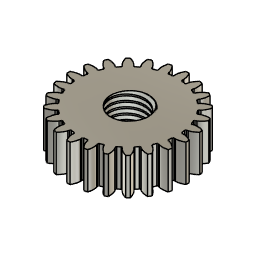
gear v1 (Autodesk Fusion 360 design; units mm, degrees)
description: Spur Gear; Module: 1.25; Num Teeth: 24; Pressure Angle: 20.0; Backlash: 0.00 mm
Autodesk Fusion 360 part; units mm, degrees
(part 1 of 3)
sketch "Sketch1" plane through (0, 0, 0) normal (0, 0, 1) x (1, 0, 0)
sketch "Sketch1 (2)" plane through (0, 0, 0) normal (0, 0, 1) x (1, 0, 0) in component "Spur Gear (24 teeth)"
  circle A0 centre (0, 0) radius 13.4492
extrude "Extrude1" add sketch "Sketch1 (2)" along normal blind 10 makes body 1 in component "Spur Gear (24 teeth)"
sketch "Sketch2" plane through (0, 0, 0) normal (0, 0, 1) x (1, 0, 0) in component "Spur Gear (24 teeth)"
  spline S0 degree 5 poles (14.0499, -1.1314) (14.0562, -1.1319) (14.0687, -1.1327) (14.0876, -1.1335) (14.1127, -1.1337) (14.1442, -1.1327) (14.1757, -1.1308) (14.2072, -1.1284) (14.2388, -1.1257) (14.2703, -1.1227) (14.3019, -1.1196) (14.3335, -1.1161) (14.3651, -1.1123) (14.3967, -1.1081) (14.4283, -1.1035) (14.4599, -1.0984) (14.4916, -1.093) (14.5232, -1.0873) (14.5548, -1.0814) (14.5864, -1.0752) (14.618, -1.0688) (14.6496, -1.0622) (14.6812, -1.0552) (14.7128, -1.048) (14.7444, -1.0406) (14.776, -1.0329) (14.8076, -1.0249) (14.8392, -1.0168) (14.8708, -1.0083) (14.9023, -0.9997) (14.9339, -0.9909) (14.9654, -0.9818) (14.997, -0.9725) (15.0285, -0.963) (15.06, -0.9533) (15.0915, -0.9434) (15.123, -0.9333) (15.1545, -0.923) (15.1859, -0.9124) (15.2174, -0.9017) (15.2488, -0.8908) (15.2802, -0.8797) (15.3116, -0.8684) (15.343, -0.8569) (15.3743, -0.8452) (15.4057, -0.8333) (15.437, -0.8213) (15.4683, -0.809) (15.4996, -0.7966) (15.5309, -0.784) (15.5621, -0.7712) (15.5934, -0.7583) (15.6246, -0.7451) (15.6558, -0.7318) (15.6869, -0.7183) (15.7181, -0.7047) (15.7492, -0.6909) (15.7803, -0.6769) (15.8114, -0.6627) (15.8425, -0.6484) (15.8735, -0.6339) (15.9045, -0.6192) (15.9355, -0.6044) (15.9664, -0.5894) (15.9974, -0.5742) (16.0283, -0.5589) (16.0592, -0.5434) (16.09, -0.5278) (16.1208, -0.512) (16.1516, -0.496) (16.1824, -0.4799) (16.207, -0.4669) (16.2254, -0.4571) (16.2377, -0.4505) (16.2438, -0.4472) knots 0 0 0 0 0 0 0.01428571 0.02857143 0.04285714 0.05714286 0.07142857 0.08571429 0.1 0.11428571 0.12857143 0.14285714 0.15714286 0.17142857 0.18571429 0.2 0.21428571 0.22857143 0.24285714 0.25714286 0.27142857 0.28571429 0.3 0.31428571 0.32857143 0.34285714 0.35714286 0.37142857 0.38571429 0.4 0.41428571 0.42857143 0.44285714 0.45714286 0.47142857 0.48571429 0.5 0.51428571 0.52857143 0.54285714 0.55714286 0.57142857 0.58571429 0.6 0.61428571 0.62857143 0.64285714 0.65714286 0.67142857 0.68571429 0.7 0.71428571 0.72857143 0.74285714 0.75714286 0.77142857 0.78571429 0.8 0.81428571 0.82857143 0.84285714 0.85714286 0.87142857 0.88571429 0.9 0.91428571 0.92857143 0.94285714 0.95714286 0.97142857 0.98571429 1 1 1 1 1 1
  spline S1 degree 5 poles (14.0499, 1.1314) (14.0562, 1.1319) (14.0687, 1.1327) (14.0876, 1.1335) (14.1127, 1.1337) (14.1442, 1.1327) (14.1757, 1.1308) (14.2072, 1.1284) (14.2388, 1.1257) (14.2703, 1.1227) (14.3019, 1.1196) (14.3335, 1.1161) (14.3651, 1.1123) (14.3967, 1.1081) (14.4283, 1.1035) (14.4599, 1.0984) (14.4916, 1.093) (14.5232, 1.0873) (14.5548, 1.0814) (14.5864, 1.0752) (14.618, 1.0688) (14.6496, 1.0622) (14.6812, 1.0552) (14.7128, 1.048) (14.7444, 1.0406) (14.776, 1.0329) (14.8076, 1.0249) (14.8392, 1.0168) (14.8708, 1.0083) (14.9023, 0.9997) (14.9339, 0.9909) (14.9654, 0.9818) (14.997, 0.9725) (15.0285, 0.963) (15.06, 0.9533) (15.0915, 0.9434) (15.123, 0.9333) (15.1545, 0.923) (15.1859, 0.9124) (15.2174, 0.9017) (15.2488, 0.8908) (15.2802, 0.8797) (15.3116, 0.8684) (15.343, 0.8569) (15.3743, 0.8452) (15.4057, 0.8333) (15.437, 0.8213) (15.4683, 0.809) (15.4996, 0.7966) (15.5309, 0.784) (15.5621, 0.7712) (15.5934, 0.7583) (15.6246, 0.7451) (15.6558, 0.7318) (15.6869, 0.7183) (15.7181, 0.7047) (15.7492, 0.6909) (15.7803, 0.6769) (15.8114, 0.6627) (15.8425, 0.6484) (15.8735, 0.6339) (15.9045, 0.6192) (15.9355, 0.6044) (15.9664, 0.5894) (15.9974, 0.5742) (16.0283, 0.5589) (16.0592, 0.5434) (16.09, 0.5278) (16.1208, 0.512) (16.1516, 0.496) (16.1824, 0.4799) (16.207, 0.4669) (16.2254, 0.4571) (16.2377, 0.4505) (16.2438, 0.4472) knots 0 0 0 0 0 0 0.01428571 0.02857143 0.04285714 0.05714286 0.07142857 0.08571429 0.1 0.11428571 0.12857143 0.14285714 0.15714286 0.17142857 0.18571429 0.2 0.21428571 0.22857143 0.24285714 0.25714286 0.27142857 0.28571429 0.3 0.31428571 0.32857143 0.34285714 0.35714286 0.37142857 0.38571429 0.4 0.41428571 0.42857143 0.44285714 0.45714286 0.47142857 0.48571429 0.5 0.51428571 0.52857143 0.54285714 0.55714286 0.57142857 0.58571429 0.6 0.61428571 0.62857143 0.64285714 0.65714286 0.67142857 0.68571429 0.7 0.71428571 0.72857143 0.74285714 0.75714286 0.77142857 0.78571429 0.8 0.81428571 0.82857143 0.84285714 0.85714286 0.87142857 0.88571429 0.9 0.91428571 0.92857143 0.94285714 0.95714286 0.97142857 0.98571429 1 1 1 1 1 1
  arc A0 (16.2438, -0.4472) -> (16.2438, 0.4472) centre (0, 0) ccw
  line L0 (13.3958, -1.0795) -> (14.0499, -1.1314)
  line L1 (13.3958, 1.0795) -> (14.0499, 1.1314)
  line L2 (13.3958, -1.0795) -> (13.3958, 1.0795)
  point P0 (14.2045, -1.1286)
  point P1 (14.3601, -1.1129)
  point P2 (14.5163, -1.0885)
  point P3 (14.673, -1.057)
  point P4 (14.8299, -1.0191)
  point P5 (14.9871, -0.9754)
  point P6 (15.1444, -0.9262)
  point P7 (15.3018, -0.8719)
  point P8 (15.4592, -0.8126)
  point P9 (15.6165, -0.7485)
  point P10 (15.7737, -0.6798)
  point P11 (15.9307, -0.6066)
  point P12 (16.0874, -0.5291)
  point P13 (14.2045, 1.1286)
  point P14 (14.3601, 1.1129)
  point P15 (14.5163, 1.0885)
  point P16 (14.673, 1.057)
  point P17 (14.8299, 1.0191)
  point P18 (14.9871, 0.9754)
  point P19 (15.1444, 0.9262)
  point P20 (15.3018, 0.8719)
  point P21 (15.4592, 0.8126)
  point P22 (15.6165, 0.7485)
  point P23 (15.7737, 0.6798)
  point P24 (15.9307, 0.6066)
  point P25 (16.0874, 0.5291)
extrude "Extrude2" add sketch "Sketch2" along normal blind 10 bodies 1 in component "Spur Gear (24 teeth)"
fillet "Fillet1" radius 0.25 2 edges at (13.4057, -1.0803, 5) (13.4057, 1.0803, 5) on bodies 1 in component "Spur Gear (24 teeth)"
pattern_circular "C-Pattern1" count 24 over 360 about axis through (0, 0, 0) along (0, 0, 1) of "Extrude2", "Fillet1" in component "Spur Gear (24 teeth)"
sketch "Sketch3" plane through (0, 0, 0) normal (0, 0, 1) x (1, 0, 0) in component "Spur Gear (24 teeth)"
  circle A0 centre (0, 0) radius 15 construction
copy_body "CopyPasteBodies1" bodies 1 makes body 2
move_body "Move1" bodies 2 to x (1, 0, 0) y (0, 1, 0) z (0, 0, 1) at (0, 40, 0)
sketch "Sketch2 (2)" plane through (0, 0, 10) normal (0, 0, 1) x (-1, 0, 0)
  arc A0 (-13.2706, -37.8154) -> (-13.3838, -38.6755) centre (0, -40) ccw
  arc A1 (-13.6524, -38.9001) -> (-13.3838, -38.6755) centre (-13.6326, -38.6509) ccw
  line L0 (-13.6524, -38.9001) -> (-14.0499, -38.8686)
  spline S0 degree 5 poles (-14.0499, -38.8686) (-14.0562, -38.8681) (-14.0687, -38.8673) (-14.0876, -38.8665) (-14.1127, -38.8663) (-14.1442, -38.8673) (-14.1757, -38.8692) (-14.2072, -38.8716) (-14.2388, -38.8743) (-14.2703, -38.8773) (-14.3019, -38.8804) (-14.3335, -38.8839) (-14.3651, -38.8877) (-14.3967, -38.8919) (-14.4283, -38.8965) (-14.4599, -38.9016) (-14.4916, -38.907) (-14.5232, -38.9127) (-14.5548, -38.9186) (-14.5864, -38.9248) (-14.618, -38.9312) (-14.6496, -38.9378) (-14.6812, -38.9448) (-14.7128, -38.952) (-14.7444, -38.9594) (-14.776, -38.9671) (-14.8076, -38.9751) (-14.8392, -38.9832) (-14.8708, -38.9917) (-14.9023, -39.0003) (-14.9339, -39.0091) (-14.9654, -39.0182) (-14.997, -39.0275) (-15.0285, -39.037) (-15.06, -39.0467) (-15.0915, -39.0566) (-15.123, -39.0667) (-15.1545, -39.077) (-15.1859, -39.0876) (-15.2174, -39.0983) (-15.2488, -39.1092) (-15.2802, -39.1203) (-15.3116, -39.1316) (-15.343, -39.1431) (-15.3743, -39.1548) (-15.4057, -39.1667) (-15.437, -39.1787) (-15.4683, -39.191) (-15.4996, -39.2034) (-15.5309, -39.216) (-15.5621, -39.2288) (-15.5934, -39.2417) (-15.6246, -39.2549) (-15.6558, -39.2682) (-15.6869, -39.2817) (-15.7181, -39.2953) (-15.7492, -39.3091) (-15.7803, -39.3231) (-15.8114, -39.3373) (-15.8425, -39.3516) (-15.8735, -39.3661) (-15.9045, -39.3808) (-15.9355, -39.3956) (-15.9664, -39.4106) (-15.9974, -39.4258) (-16.0283, -39.4411) (-16.0592, -39.4566) (-16.09, -39.4722) (-16.1208, -39.488) (-16.1516, -39.504) (-16.1824, -39.5201) (-16.207, -39.5331) (-16.2254, -39.5429) (-16.2377, -39.5495) (-16.2438, -39.5528) knots 0 0 0 0 0 0 0.01428571 0.02857143 0.04285714 0.05714286 0.07142857 0.08571429 0.1 0.11428571 0.12857143 0.14285714 0.15714286 0.17142857 0.18571429 0.2 0.21428571 0.22857143 0.24285714 0.25714286 0.27142857 0.28571429 0.3 0.31428571 0.32857143 0.34285714 0.35714286 0.37142857 0.38571429 0.4 0.41428571 0.42857143 0.44285714 0.45714286 0.47142857 0.48571429 0.5 0.51428571 0.52857143 0.54285714 0.55714286 0.57142857 0.58571429 0.6 0.61428571 0.62857143 0.64285714 0.65714286 0.67142857 0.68571429 0.7 0.71428571 0.72857143 0.74285714 0.75714286 0.77142857 0.78571429 0.8 0.81428571 0.82857143 0.84285714 0.85714286 0.87142857 0.88571429 0.9 0.91428571 0.92857143 0.94285714 0.95714286 0.97142857 0.98571429 1 1 1 1 1 1
  arc A2 (-16.2438, -39.5528) -> (-16.2438, -40.4472) centre (0, -40) ccw
  spline S1 degree 5 poles (-16.2438, -40.4472) (-16.2377, -40.4505) (-16.2254, -40.4571) (-16.207, -40.4669) (-16.1824, -40.4799) (-16.1516, -40.496) (-16.1208, -40.512) (-16.09, -40.5278) (-16.0592, -40.5434) (-16.0283, -40.5589) (-15.9974, -40.5742) (-15.9664, -40.5894) (-15.9355, -40.6044) (-15.9045, -40.6192) (-15.8735, -40.6339) (-15.8425, -40.6484) (-15.8114, -40.6627) (-15.7803, -40.6769) (-15.7492, -40.6909) (-15.7181, -40.7047) (-15.6869, -40.7183) (-15.6558, -40.7318) (-15.6246, -40.7451) (-15.5934, -40.7583) (-15.5621, -40.7712) (-15.5309, -40.784) (-15.4996, -40.7966) (-15.4683, -40.809) (-15.437, -40.8213) (-15.4057, -40.8333) (-15.3743, -40.8452) (-15.343, -40.8569) (-15.3116, -40.8684) (-15.2802, -40.8797) (-15.2488, -40.8908) (-15.2174, -40.9017) (-15.1859, -40.9124) (-15.1545, -40.923) (-15.123, -40.9333) (-15.0915, -40.9434) (-15.06, -40.9533) (-15.0285, -40.963) (-14.997, -40.9725) (-14.9654, -40.9818) (-14.9339, -40.9909) (-14.9023, -40.9997) (-14.8708, -41.0083) (-14.8392, -41.0168) (-14.8076, -41.0249) (-14.776, -41.0329) (-14.7444, -41.0406) (-14.7128, -41.048) (-14.6812, -41.0552) (-14.6496, -41.0622) (-14.618, -41.0688) (-14.5864, -41.0752) (-14.5548, -41.0814) (-14.5232, -41.0873) (-14.4916, -41.093) (-14.4599, -41.0984) (-14.4283, -41.1035) (-14.3967, -41.1081) (-14.3651, -41.1123) (-14.3335, -41.1161) (-14.3019, -41.1196) (-14.2703, -41.1227) (-14.2388, -41.1257) (-14.2072, -41.1284) (-14.1757, -41.1308) (-14.1442, -41.1327) (-14.1127, -41.1337) (-14.0876, -41.1335) (-14.0687, -41.1327) (-14.0562, -41.1319) (-14.0499, -41.1314) knots -1 -1 -1 -1 -1 -1 -0.98571429 -0.97142857 -0.95714286 -0.94285714 -0.92857143 -0.91428571 -0.9 -0.88571429 -0.87142857 -0.85714286 -0.84285714 -0.82857143 -0.81428571 -0.8 -0.78571429 -0.77142857 -0.75714286 -0.74285714 -0.72857143 -0.71428571 -0.7 -0.68571429 -0.67142857 -0.65714286 -0.64285714 -0.62857143 -0.61428571 -0.6 -0.58571429 -0.57142857 -0.55714286 -0.54285714 -0.52857143 -0.51428571 -0.5 -0.48571429 -0.47142857 -0.45714286 -0.44285714 -0.42857143 -0.41428571 -0.4 -0.38571429 -0.37142857 -0.35714286 -0.34285714 -0.32857143 -0.31428571 -0.3 -0.28571429 -0.27142857 -0.25714286 -0.24285714 -0.22857143 -0.21428571 -0.2 -0.18571429 -0.17142857 -0.15714286 -0.14285714 -0.12857143 -0.11428571 -0.1 -0.08571429 -0.07142857 -0.05714286 -0.04285714 -0.02857143 -0.01428571 0 0 0 0 0 0
  line L1 (-14.0499, -41.1314) -> (-13.6524, -41.0999)
  arc A3 (-13.3838, -41.3245) -> (-13.6524, -41.0999) centre (-13.6326, -41.3491) ccw
  arc A4 (-13.3838, -41.3245) -> (-13.2706, -42.1846) centre (0, -40) ccw
  arc A5 (-13.4718, -42.4711) -> (-13.2706, -42.1846) centre (-13.5173, -42.2252) ccw
  line L2 (-13.4718, -42.4711) -> (-13.864, -42.5435)
  spline S2 degree 5 poles (-13.864, -42.5435) (-13.8702, -42.5447) (-13.8825, -42.5471) (-13.9009, -42.5512) (-13.9253, -42.5576) (-13.9554, -42.5667) (-13.9854, -42.5766) (-14.0152, -42.5871) (-14.0449, -42.5979) (-14.0747, -42.609) (-14.1044, -42.6202) (-14.134, -42.6317) (-14.1635, -42.6435) (-14.193, -42.6558) (-14.2223, -42.6685) (-14.2515, -42.6815) (-14.2807, -42.6949) (-14.3097, -42.7086) (-14.3387, -42.7225) (-14.3677, -42.7367) (-14.3966, -42.751) (-14.4254, -42.7656) (-14.4541, -42.7805) (-14.4828, -42.7956) (-14.5114, -42.811) (-14.5399, -42.8266) (-14.5683, -42.8425) (-14.5967, -42.8586) (-14.625, -42.8749) (-14.6533, -42.8914) (-14.6815, -42.9081) (-14.7096, -42.925) (-14.7377, -42.9421) (-14.7657, -42.9594) (-14.7936, -42.977) (-14.8214, -42.9947) (-14.8492, -43.0126) (-14.877, -43.0307) (-14.9046, -43.0491) (-14.9322, -43.0675) (-14.9597, -43.0862) (-14.9872, -43.1051) (-15.0146, -43.1241) (-15.042, -43.1434) (-15.0692, -43.1628) (-15.0964, -43.1823) (-15.1236, -43.2021) (-15.1506, -43.222) (-15.1777, -43.2421) (-15.2046, -43.2624) (-15.2315, -43.2828) (-15.2583, -43.3034) (-15.285, -43.3242) (-15.3117, -43.3451) (-15.3383, -43.3662) (-15.3649, -43.3875) (-15.3914, -43.4089) (-15.4178, -43.4304) (-15.4442, -43.4522) (-15.4704, -43.4741) (-15.4967, -43.4961) (-15.5228, -43.5183) (-15.5489, -43.5406) (-15.5749, -43.5631) (-15.6009, -43.5858) (-15.6268, -43.6086) (-15.6526, -43.6315) (-15.6784, -43.6546) (-15.704, -43.6779) (-15.7297, -43.7012) (-15.7552, -43.7248) (-15.7756, -43.7437) (-15.7908, -43.758) (-15.801, -43.7675) (-15.8061, -43.7723) knots 0 0 0 0 0 0 0.01428571 0.02857143 0.04285714 0.05714286 0.07142857 0.08571429 0.1 0.11428571 0.12857143 0.14285714 0.15714286 0.17142857 0.18571429 0.2 0.21428571 0.22857143 0.24285714 0.25714286 0.27142857 0.28571429 0.3 0.31428571 0.32857143 0.34285714 0.35714286 0.37142857 0.38571429 0.4 0.41428571 0.42857143 0.44285714 0.45714286 0.47142857 0.48571429 0.5 0.51428571 0.52857143 0.54285714 0.55714286 0.57142857 0.58571429 0.6 0.61428571 0.62857143 0.64285714 0.65714286 0.67142857 0.68571429 0.7 0.71428571 0.72857143 0.74285714 0.75714286 0.77142857 0.78571429 0.8 0.81428571 0.82857143 0.84285714 0.85714286 0.87142857 0.88571429 0.9 0.91428571 0.92857143 0.94285714 0.95714286 0.97142857 0.98571429 1 1 1 1 1 1
  arc A6 (-15.8061, -43.7723) -> (-15.5746, -44.6361) centre (0, -40) ccw
  spline S3 degree 5 poles (-15.5746, -44.6361) (-15.5678, -44.6377) (-15.5543, -44.6409) (-15.5339, -44.6457) (-15.5068, -44.6519) (-15.4729, -44.6595) (-15.439, -44.6669) (-15.4052, -44.6742) (-15.3713, -44.6813) (-15.3375, -44.6883) (-15.3037, -44.6951) (-15.2699, -44.7017) (-15.2361, -44.7082) (-15.2023, -44.7145) (-15.1686, -44.7206) (-15.1348, -44.7266) (-15.1011, -44.7324) (-15.0674, -44.738) (-15.0338, -44.7435) (-15.0001, -44.7488) (-14.9665, -44.754) (-14.9329, -44.7589) (-14.8993, -44.7637) (-14.8658, -44.7683) (-14.8323, -44.7727) (-14.7988, -44.777) (-14.7653, -44.7811) (-14.7319, -44.785) (-14.6984, -44.7887) (-14.6651, -44.7922) (-14.6317, -44.7956) (-14.5984, -44.7987) (-14.5651, -44.8017) (-14.5319, -44.8045) (-14.4986, -44.8071) (-14.4655, -44.8095) (-14.4323, -44.8118) (-14.3992, -44.8138) (-14.3661, -44.8156) (-14.3331, -44.8172) (-14.3001, -44.8187) (-14.2672, -44.8199) (-14.2342, -44.8209) (-14.2014, -44.8217) (-14.1686, -44.8223) (-14.1358, -44.8227) (-14.1031, -44.8228) (-14.0704, -44.8228) (-14.0378, -44.8225) (-14.0052, -44.822) (-13.9727, -44.8213) (-13.9403, -44.8203) (-13.9079, -44.8191) (-13.8756, -44.8176) (-13.8433, -44.8158) (-13.8111, -44.8138) (-13.779, -44.8116) (-13.7469, -44.8092) (-13.7149, -44.8065) (-13.6829, -44.8035) (-13.6511, -44.8002) (-13.6194, -44.7965) (-13.5877, -44.7924) (-13.5562, -44.7879) (-13.5248, -44.783) (-13.4935, -44.7779) (-13.4623, -44.7726) (-13.4311, -44.7671) (-13.4, -44.7613) (-13.3691, -44.7549) (-13.3384, -44.7477) (-13.3142, -44.741) (-13.2962, -44.7354) (-13.2843, -44.7313) (-13.2783, -44.7292) knots -1 -1 -1 -1 -1 -1 -0.98571429 -0.97142857 -0.95714286 -0.94285714 -0.92857143 -0.91428571 -0.9 -0.88571429 -0.87142857 -0.85714286 -0.84285714 -0.82857143 -0.81428571 -0.8 -0.78571429 -0.77142857 -0.75714286 -0.74285714 -0.72857143 -0.71428571 -0.7 -0.68571429 -0.67142857 -0.65714286 -0.64285714 -0.62857143 -0.61428571 -0.6 -0.58571429 -0.57142857 -0.55714286 -0.54285714 -0.52857143 -0.51428571 -0.5 -0.48571429 -0.47142857 -0.45714286 -0.44285714 -0.42857143 -0.41428571 -0.4 -0.38571429 -0.37142857 -0.35714286 -0.34285714 -0.32857143 -0.31428571 -0.3 -0.28571429 -0.27142857 -0.25714286 -0.24285714 -0.22857143 -0.21428571 -0.2 -0.18571429 -0.17142857 -0.15714286 -0.14285714 -0.12857143 -0.11428571 -0.1 -0.08571429 -0.07142857 -0.05714286 -0.04285714 -0.02857143 -0.01428571 0 0 0 0 0 0
  line L3 (-13.2783, -44.7292) -> (-12.9025, -44.5959)
  arc A7 (-12.585, -44.7433) -> (-12.9025, -44.5959) centre (-12.8189, -44.8315) ccw
  arc A8 (-12.585, -44.7433) -> (-12.253, -45.5449) centre (0, -40) ccw
  arc A9 (-12.3732, -45.8737) -> (-12.253, -45.5449) centre (-12.4807, -45.648) ccw
  line L4 (-12.3732, -45.8737) -> (-12.7333, -46.0451)
  spline S4 degree 5 poles (-12.7333, -46.0451) (-12.739, -46.0478) (-12.7503, -46.0534) (-12.767, -46.0621) (-12.7888, -46.0745) (-12.8156, -46.0911) (-12.8419, -46.1085) (-12.868, -46.1264) (-12.894, -46.1445) (-12.9198, -46.1629) (-12.9456, -46.1814) (-12.9713, -46.2002) (-12.9967, -46.2193) (-13.022, -46.2387) (-13.047, -46.2585) (-13.0719, -46.2787) (-13.0966, -46.2992) (-13.1211, -46.3199) (-13.1455, -46.3409) (-13.1698, -46.362) (-13.194, -46.3834) (-13.218, -46.405) (-13.2419, -46.4268) (-13.2657, -46.4488) (-13.2894, -46.471) (-13.3129, -46.4935) (-13.3362, -46.5162) (-13.3595, -46.5391) (-13.3826, -46.5621) (-13.4057, -46.5854) (-13.4286, -46.6088) (-13.4514, -46.6324) (-13.474, -46.6562) (-13.4966, -46.6802) (-13.519, -46.7044) (-13.5413, -46.7287) (-13.5635, -46.7532) (-13.5856, -46.7779) (-13.6076, -46.8028) (-13.6295, -46.8278) (-13.6512, -46.8529) (-13.6729, -46.8783) (-13.6944, -46.9038) (-13.7158, -46.9294) (-13.7372, -46.9552) (-13.7584, -46.9812) (-13.7795, -47.0073) (-13.8005, -47.0335) (-13.8214, -47.0599) (-13.8422, -47.0865) (-13.8628, -47.1132) (-13.8834, -47.14) (-13.9039, -47.167) (-13.9242, -47.1941) (-13.9445, -47.2214) (-13.9646, -47.2488) (-13.9847, -47.2763) (-14.0046, -47.304) (-14.0244, -47.3318) (-14.0442, -47.3597) (-14.0638, -47.3878) (-14.0833, -47.416) (-14.1027, -47.4443) (-14.122, -47.4728) (-14.1412, -47.5014) (-14.1603, -47.5301) (-14.1793, -47.559) (-14.1982, -47.5879) (-14.217, -47.617) (-14.2357, -47.6463) (-14.2543, -47.6756) (-14.2691, -47.6992) (-14.2802, -47.7169) (-14.2875, -47.7287) (-14.2912, -47.7347) knots 0 0 0 0 0 0 0.01428571 0.02857143 0.04285714 0.05714286 0.07142857 0.08571429 0.1 0.11428571 0.12857143 0.14285714 0.15714286 0.17142857 0.18571429 0.2 0.21428571 0.22857143 0.24285714 0.25714286 0.27142857 0.28571429 0.3 0.31428571 0.32857143 0.34285714 0.35714286 0.37142857 0.38571429 0.4 0.41428571 0.42857143 0.44285714 0.45714286 0.47142857 0.48571429 0.5 0.51428571 0.52857143 0.54285714 0.55714286 0.57142857 0.58571429 0.6 0.61428571 0.62857143 0.64285714 0.65714286 0.67142857 0.68571429 0.7 0.71428571 0.72857143 0.74285714 0.75714286 0.77142857 0.78571429 0.8 0.81428571 0.82857143 0.84285714 0.85714286 0.87142857 0.88571429 0.9 0.91428571 0.92857143 0.94285714 0.95714286 0.97142857 0.98571429 1 1 1 1 1 1
  arc A10 (-14.2912, -47.7347) -> (-13.844, -48.5092) centre (0, -40) ccw
  spline S5 degree 5 poles (-13.844, -48.5092) (-13.837, -48.509) (-13.8231, -48.5085) (-13.8022, -48.5078) (-13.7744, -48.5068) (-13.7397, -48.5054) (-13.7051, -48.5038) (-13.6705, -48.5021) (-13.6359, -48.5002) (-13.6014, -48.4982) (-13.567, -48.496) (-13.5327, -48.4936) (-13.4983, -48.4911) (-13.4641, -48.4885) (-13.4299, -48.4857) (-13.3958, -48.4827) (-13.3617, -48.4796) (-13.3277, -48.4763) (-13.2938, -48.4729) (-13.2599, -48.4693) (-13.2261, -48.4656) (-13.1924, -48.4617) (-13.1587, -48.4576) (-13.1251, -48.4534) (-13.0916, -48.449) (-13.0581, -48.4444) (-13.0248, -48.4397) (-12.9914, -48.4348) (-12.9582, -48.4298) (-12.925, -48.4245) (-12.892, -48.4191) (-12.859, -48.4136) (-12.826, -48.4078) (-12.7932, -48.4019) (-12.7604, -48.3958) (-12.7278, -48.3896) (-12.6952, -48.3832) (-12.6627, -48.3765) (-12.6302, -48.3697) (-12.5979, -48.3628) (-12.5657, -48.3556) (-12.5335, -48.3483) (-12.5015, -48.3407) (-12.4695, -48.333) (-12.4377, -48.3251) (-12.4059, -48.3169) (-12.3743, -48.3086) (-12.3428, -48.3001) (-12.3113, -48.2914) (-12.28, -48.2825) (-12.2488, -48.2734) (-12.2177, -48.2641) (-12.1867, -48.2545) (-12.1559, -48.2447) (-12.1252, -48.2346) (-12.0946, -48.2244) (-12.0641, -48.2139) (-12.0338, -48.2032) (-12.0035, -48.1924) (-11.9735, -48.1812) (-11.9436, -48.1698) (-11.9139, -48.158) (-11.8844, -48.1459) (-11.8551, -48.1334) (-11.826, -48.1205) (-11.7971, -48.1075) (-11.7683, -48.0943) (-11.7396, -48.0808) (-11.7111, -48.0672) (-11.6829, -48.0531) (-11.6551, -48.0382) (-11.6334, -48.0255) (-11.6175, -48.0154) (-11.6071, -48.0083) (-11.6019, -48.0048) knots -1 -1 -1 -1 -1 -1 -0.98571429 -0.97142857 -0.95714286 -0.94285714 -0.92857143 -0.91428571 -0.9 -0.88571429 -0.87142857 -0.85714286 -0.84285714 -0.82857143 -0.81428571 -0.8 -0.78571429 -0.77142857 -0.75714286 -0.74285714 -0.72857143 -0.71428571 -0.7 -0.68571429 -0.67142857 -0.65714286 -0.64285714 -0.62857143 -0.61428571 -0.6 -0.58571429 -0.57142857 -0.55714286 -0.54285714 -0.52857143 -0.51428571 -0.5 -0.48571429 -0.47142857 -0.45714286 -0.44285714 -0.42857143 -0.41428571 -0.4 -0.38571429 -0.37142857 -0.35714286 -0.34285714 -0.32857143 -0.31428571 -0.3 -0.28571429 -0.27142857 -0.25714286 -0.24285714 -0.22857143 -0.21428571 -0.2 -0.18571429 -0.17142857 -0.15714286 -0.14285714 -0.12857143 -0.11428571 -0.1 -0.08571429 -0.07142857 -0.05714286 -0.04285714 -0.02857143 -0.01428571 0 0 0 0 0 0
  line L5 (-11.6019, -48.0048) -> (-11.2734, -47.7787)
  arc A11 (-10.9285, -47.8389) -> (-11.2734, -47.7787) centre (-11.1316, -47.9847) ccw
  arc A12 (-10.9285, -47.8389) -> (-10.4003, -48.5272) centre (0, -40) ccw
  arc A13 (-10.4314, -48.876) -> (-10.4003, -48.5272) centre (-10.5937, -48.6858) ccw
  line L6 (-10.4314, -48.876) -> (-10.7348, -49.1348)
  spline S6 degree 5 poles (-10.7348, -49.1348) (-10.7396, -49.1388) (-10.7491, -49.1471) (-10.7629, -49.1599) (-10.7809, -49.1775) (-10.8024, -49.2005) (-10.8234, -49.2241) (-10.8439, -49.2481) (-10.8643, -49.2724) (-10.8845, -49.2968) (-10.9046, -49.3213) (-10.9245, -49.3461) (-10.9442, -49.3711) (-10.9636, -49.3965) (-10.9826, -49.4221) (-11.0014, -49.448) (-11.02, -49.4742) (-11.0383, -49.5006) (-11.0565, -49.5271) (-11.0744, -49.5539) (-11.0923, -49.5807) (-11.1099, -49.6078) (-11.1274, -49.635) (-11.1446, -49.6625) (-11.1617, -49.6901) (-11.1786, -49.7179) (-11.1953, -49.7458) (-11.2119, -49.7739) (-11.2282, -49.8022) (-11.2444, -49.8306) (-11.2605, -49.8592) (-11.2764, -49.8879) (-11.2921, -49.9168) (-11.3077, -49.9458) (-11.3231, -49.9749) (-11.3384, -50.0042) (-11.3535, -50.0336) (-11.3685, -50.0632) (-11.3833, -50.0929) (-11.3979, -50.1227) (-11.4124, -50.1526) (-11.4268, -50.1827) (-11.441, -50.2129) (-11.455, -50.2432) (-11.4689, -50.2736) (-11.4827, -50.3042) (-11.4963, -50.3349) (-11.5098, -50.3657) (-11.5232, -50.3966) (-11.5364, -50.4276) (-11.5494, -50.4588) (-11.5624, -50.49) (-11.5751, -50.5214) (-11.5878, -50.5528) (-11.6003, -50.5844) (-11.6127, -50.6161) (-11.6249, -50.6479) (-11.637, -50.6798) (-11.6489, -50.7118) (-11.6608, -50.7438) (-11.6725, -50.776) (-11.684, -50.8083) (-11.6954, -50.8407) (-11.7067, -50.8732) (-11.7179, -50.9058) (-11.7289, -50.9385) (-11.7398, -50.9713) (-11.7505, -51.0042) (-11.7612, -51.0371) (-11.7717, -51.0702) (-11.782, -51.1033) (-11.7902, -51.1299) (-11.7963, -51.1499) (-11.8003, -51.1633) (-11.8023, -51.1699) knots 0 0 0 0 0 0 0.01428571 0.02857143 0.04285714 0.05714286 0.07142857 0.08571429 0.1 0.11428571 0.12857143 0.14285714 0.15714286 0.17142857 0.18571429 0.2 0.21428571 0.22857143 0.24285714 0.25714286 0.27142857 0.28571429 0.3 0.31428571 0.32857143 0.34285714 0.35714286 0.37142857 0.38571429 0.4 0.41428571 0.42857143 0.44285714 0.45714286 0.47142857 0.48571429 0.5 0.51428571 0.52857143 0.54285714 0.55714286 0.57142857 0.58571429 0.6 0.61428571 0.62857143 0.64285714 0.65714286 0.67142857 0.68571429 0.7 0.71428571 0.72857143 0.74285714 0.75714286 0.77142857 0.78571429 0.8 0.81428571 0.82857143 0.84285714 0.85714286 0.87142857 0.88571429 0.9 0.91428571 0.92857143 0.94285714 0.95714286 0.97142857 0.98571429 1 1 1 1 1 1
  arc A14 (-11.8023, -51.1699) -> (-11.1699, -51.8023) centre (0, -40) ccw
  spline S7 degree 5 poles (-11.1699, -51.8023) (-11.1633, -51.8003) (-11.1499, -51.7963) (-11.1299, -51.7902) (-11.1033, -51.782) (-11.0702, -51.7717) (-11.0371, -51.7612) (-11.0042, -51.7505) (-10.9713, -51.7398) (-10.9385, -51.7289) (-10.9058, -51.7179) (-10.8732, -51.7067) (-10.8407, -51.6954) (-10.8083, -51.684) (-10.776, -51.6725) (-10.7438, -51.6608) (-10.7118, -51.6489) (-10.6798, -51.637) (-10.6479, -51.6249) (-10.6161, -51.6127) (-10.5844, -51.6003) (-10.5528, -51.5878) (-10.5214, -51.5751) (-10.49, -51.5624) (-10.4588, -51.5494) (-10.4276, -51.5364) (-10.3966, -51.5232) (-10.3657, -51.5098) (-10.3349, -51.4963) (-10.3042, -51.4827) (-10.2736, -51.4689) (-10.2432, -51.455) (-10.2129, -51.441) (-10.1827, -51.4268) (-10.1526, -51.4124) (-10.1227, -51.3979) (-10.0929, -51.3833) (-10.0632, -51.3685) (-10.0336, -51.3535) (-10.0042, -51.3384) (-9.9749, -51.3231) (-9.9458, -51.3077) (-9.9168, -51.2921) (-9.8879, -51.2764) (-9.8592, -51.2605) (-9.8306, -51.2444) (-9.8022, -51.2282) (-9.7739, -51.2119) (-9.7458, -51.1953) (-9.7179, -51.1786) (-9.6901, -51.1617) (-9.6625, -51.1446) (-9.635, -51.1274) (-9.6078, -51.1099) (-9.5807, -51.0923) (-9.5539, -51.0744) (-9.5271, -51.0565) (-9.5006, -51.0383) (-9.4742, -51.02) (-9.448, -51.0014) (-9.4221, -50.9826) (-9.3965, -50.9636) (-9.3711, -50.9442) (-9.3461, -50.9245) (-9.3213, -50.9046) (-9.2968, -50.8845) (-9.2724, -50.8643) (-9.2481, -50.8439) (-9.2241, -50.8234) (-9.2005, -50.8024) (-9.1775, -50.7809) (-9.1599, -50.7629) (-9.1471, -50.7491) (-9.1388, -50.7396) (-9.1348, -50.7348) knots -1 -1 -1 -1 -1 -1 -0.98571429 -0.97142857 -0.95714286 -0.94285714 -0.92857143 -0.91428571 -0.9 -0.88571429 -0.87142857 -0.85714286 -0.84285714 -0.82857143 -0.81428571 -0.8 -0.78571429 -0.77142857 -0.75714286 -0.74285714 -0.72857143 -0.71428571 -0.7 -0.68571429 -0.67142857 -0.65714286 -0.64285714 -0.62857143 -0.61428571 -0.6 -0.58571429 -0.57142857 -0.55714286 -0.54285714 -0.52857143 -0.51428571 -0.5 -0.48571429 -0.47142857 -0.45714286 -0.44285714 -0.42857143 -0.41428571 -0.4 -0.38571429 -0.37142857 -0.35714286 -0.34285714 -0.32857143 -0.31428571 -0.3 -0.28571429 -0.27142857 -0.25714286 -0.24285714 -0.22857143 -0.21428571 -0.2 -0.18571429 -0.17142857 -0.15714286 -0.14285714 -0.12857143 -0.11428571 -0.1 -0.08571429 -0.07142857 -0.05714286 -0.04285714 -0.02857143 -0.01428571 0 0 0 0 0 0
  line L7 (-9.1348, -50.7348) -> (-8.876, -50.4314)
  arc A15 (-8.5272, -50.4003) -> (-8.876, -50.4314) centre (-8.6858, -50.5937) ccw
  arc A16 (-8.5272, -50.4003) -> (-7.8389, -50.9285) centre (0, -40) ccw
  arc A17 (-7.7787, -51.2734) -> (-7.8389, -50.9285) centre (-7.9847, -51.1316) ccw
  line L8 (-7.7787, -51.2734) -> (-8.0048, -51.6019)
  spline S8 degree 5 poles (-8.0048, -51.6019) (-8.0083, -51.6071) (-8.0154, -51.6175) (-8.0255, -51.6334) (-8.0382, -51.6551) (-8.0531, -51.6829) (-8.0672, -51.7111) (-8.0808, -51.7396) (-8.0943, -51.7683) (-8.1075, -51.7971) (-8.1205, -51.826) (-8.1334, -51.8551) (-8.1459, -51.8844) (-8.158, -51.9139) (-8.1698, -51.9436) (-8.1812, -51.9735) (-8.1924, -52.0035) (-8.2032, -52.0338) (-8.2139, -52.0641) (-8.2244, -52.0946) (-8.2346, -52.1252) (-8.2447, -52.1559) (-8.2545, -52.1867) (-8.2641, -52.2177) (-8.2734, -52.2488) (-8.2825, -52.28) (-8.2914, -52.3113) (-8.3001, -52.3428) (-8.3086, -52.3743) (-8.3169, -52.4059) (-8.3251, -52.4377) (-8.333, -52.4695) (-8.3407, -52.5015) (-8.3483, -52.5335) (-8.3556, -52.5657) (-8.3628, -52.5979) (-8.3697, -52.6302) (-8.3765, -52.6627) (-8.3832, -52.6952) (-8.3896, -52.7278) (-8.3958, -52.7604) (-8.4019, -52.7932) (-8.4078, -52.826) (-8.4136, -52.859) (-8.4191, -52.892) (-8.4245, -52.925) (-8.4298, -52.9582) (-8.4348, -52.9914) (-8.4397, -53.0248) (-8.4444, -53.0581) (-8.449, -53.0916) (-8.4534, -53.1251) (-8.4576, -53.1587) (-8.4617, -53.1924) (-8.4656, -53.2261) (-8.4693, -53.2599) (-8.4729, -53.2938) (-8.4763, -53.3277) (-8.4796, -53.3617) (-8.4827, -53.3958) (-8.4857, -53.4299) (-8.4885, -53.4641) (-8.4911, -53.4983) (-8.4936, -53.5327) (-8.496, -53.567) (-8.4982, -53.6014) (-8.5002, -53.6359) (-8.5021, -53.6705) (-8.5038, -53.7051) (-8.5054, -53.7397) (-8.5068, -53.7744) (-8.5078, -53.8022) (-8.5085, -53.8231) (-8.509, -53.837) (-8.5092, -53.844) knots 0 0 0 0 0 0 0.01428571 0.02857143 0.04285714 0.05714286 0.07142857 0.08571429 0.1 0.11428571 0.12857143 0.14285714 0.15714286 0.17142857 0.18571429 0.2 0.21428571 0.22857143 0.24285714 0.25714286 0.27142857 0.28571429 0.3 0.31428571 0.32857143 0.34285714 0.35714286 0.37142857 0.38571429 0.4 0.41428571 0.42857143 0.44285714 0.45714286 0.47142857 0.48571429 0.5 0.51428571 0.52857143 0.54285714 0.55714286 0.57142857 0.58571429 0.6 0.61428571 0.62857143 0.64285714 0.65714286 0.67142857 0.68571429 0.7 0.71428571 0.72857143 0.74285714 0.75714286 0.77142857 0.78571429 0.8 0.81428571 0.82857143 0.84285714 0.85714286 0.87142857 0.88571429 0.9 0.91428571 0.92857143 0.94285714 0.95714286 0.97142857 0.98571429 1 1 1 1 1 1
  arc A18 (-8.5092, -53.844) -> (-7.7347, -54.2912) centre (0, -40) ccw
  spline S9 degree 5 poles (-7.7347, -54.2912) (-7.7287, -54.2875) (-7.7169, -54.2802) (-7.6992, -54.2691) (-7.6756, -54.2543) (-7.6463, -54.2357) (-7.617, -54.217) (-7.5879, -54.1982) (-7.559, -54.1793) (-7.5301, -54.1603) (-7.5014, -54.1412) (-7.4728, -54.122) (-7.4443, -54.1027) (-7.416, -54.0833) (-7.3878, -54.0638) (-7.3597, -54.0442) (-7.3318, -54.0244) (-7.304, -54.0046) (-7.2763, -53.9847) (-7.2488, -53.9646) (-7.2214, -53.9445) (-7.1941, -53.9242) (-7.167, -53.9039) (-7.14, -53.8834) (-7.1132, -53.8628) (-7.0865, -53.8422) (-7.0599, -53.8214) (-7.0335, -53.8005) (-7.0073, -53.7795) (-6.9812, -53.7584) (-6.9552, -53.7372) (-6.9294, -53.7158) (-6.9038, -53.6944) (-6.8783, -53.6729) (-6.8529, -53.6512) (-6.8278, -53.6295) (-6.8028, -53.6076) (-6.7779, -53.5856) (-6.7532, -53.5635) (-6.7287, -53.5413) (-6.7044, -53.519) (-6.6802, -53.4966) (-6.6562, -53.474) (-6.6324, -53.4514) (-6.6088, -53.4286) (-6.5854, -53.4057) (-6.5621, -53.3826) (-6.5391, -53.3595) (-6.5162, -53.3362) (-6.4935, -53.3129) (-6.471, -53.2894) (-6.4488, -53.2657) (-6.4268, -53.2419) (-6.405, -53.218) (-6.3834, -53.194) (-6.362, -53.1698) (-6.3409, -53.1455) (-6.3199, -53.1211) (-6.2992, -53.0966) (-6.2787, -53.0719) (-6.2585, -53.047) (-6.2387, -53.022) (-6.2193, -52.9967) (-6.2002, -52.9713) (-6.1814, -52.9456) (-6.1629, -52.9198) (-6.1445, -52.894) (-6.1264, -52.868) (-6.1085, -52.8419) (-6.0911, -52.8156) (-6.0745, -52.7888) (-6.0621, -52.767) (-6.0534, -52.7503) (-6.0478, -52.739) (-6.0451, -52.7333) knots -1 -1 -1 -1 -1 -1 -0.98571429 -0.97142857 -0.95714286 -0.94285714 -0.92857143 -0.91428571 -0.9 -0.88571429 -0.87142857 -0.85714286 -0.84285714 -0.82857143 -0.81428571 -0.8 -0.78571429 -0.77142857 -0.75714286 -0.74285714 -0.72857143 -0.71428571 -0.7 -0.68571429 -0.67142857 -0.65714286 -0.64285714 -0.62857143 -0.61428571 -0.6 -0.58571429 -0.57142857 -0.55714286 -0.54285714 -0.52857143 -0.51428571 -0.5 -0.48571429 -0.47142857 -0.45714286 -0.44285714 -0.42857143 -0.41428571 -0.4 -0.38571429 -0.37142857 -0.35714286 -0.34285714 -0.32857143 -0.31428571 -0.3 -0.28571429 -0.27142857 -0.25714286 -0.24285714 -0.22857143 -0.21428571 -0.2 -0.18571429 -0.17142857 -0.15714286 -0.14285714 -0.12857143 -0.11428571 -0.1 -0.08571429 -0.07142857 -0.05714286 -0.04285714 -0.02857143 -0.01428571 0 0 0 0 0 0
  line L9 (-6.0451, -52.7333) -> (-5.8737, -52.3732)
  arc A19 (-5.5449, -52.253) -> (-5.8737, -52.3732) centre (-5.648, -52.4807) ccw
  arc A20 (-5.5449, -52.253) -> (-4.7433, -52.585) centre (0, -40) ccw
  arc A21 (-4.5959, -52.9025) -> (-4.7433, -52.585) centre (-4.8315, -52.8189) ccw
  line L10 (-4.5959, -52.9025) -> (-4.7292, -53.2783)
  spline S10 degree 5 poles (-4.7292, -53.2783) (-4.7313, -53.2843) (-4.7354, -53.2962) (-4.741, -53.3142) (-4.7477, -53.3384) (-4.7549, -53.3691) (-4.7613, -53.4) (-4.7671, -53.4311) (-4.7726, -53.4623) (-4.7779, -53.4935) (-4.783, -53.5248) (-4.7879, -53.5562) (-4.7924, -53.5877) (-4.7965, -53.6194) (-4.8002, -53.6511) (-4.8035, -53.6829) (-4.8065, -53.7149) (-4.8092, -53.7469) (-4.8116, -53.779) (-4.8138, -53.8111) (-4.8158, -53.8433) (-4.8176, -53.8756) (-4.8191, -53.9079) (-4.8203, -53.9403) (-4.8213, -53.9727) (-4.822, -54.0052) (-4.8225, -54.0378) (-4.8228, -54.0704) (-4.8228, -54.1031) (-4.8227, -54.1358) (-4.8223, -54.1686) (-4.8217, -54.2014) (-4.8209, -54.2342) (-4.8199, -54.2672) (-4.8187, -54.3001) (-4.8172, -54.3331) (-4.8156, -54.3661) (-4.8138, -54.3992) (-4.8118, -54.4323) (-4.8095, -54.4655) (-4.8071, -54.4986) (-4.8045, -54.5319) (-4.8017, -54.5651) (-4.7987, -54.5984) (-4.7956, -54.6317) (-4.7922, -54.6651) (-4.7887, -54.6984) (-4.785, -54.7319) (-4.7811, -54.7653) (-4.777, -54.7988) (-4.7727, -54.8323) (-4.7683, -54.8658) (-4.7637, -54.8993) (-4.7589, -54.9329) (-4.754, -54.9665) (-4.7488, -55.0001) (-4.7435, -55.0338) (-4.738, -55.0674) (-4.7324, -55.1011) (-4.7266, -55.1348) (-4.7206, -55.1686) (-4.7145, -55.2023) (-4.7082, -55.2361) (-4.7017, -55.2699) (-4.6951, -55.3037) (-4.6883, -55.3375) (-4.6813, -55.3713) (-4.6742, -55.4052) (-4.6669, -55.439) (-4.6595, -55.4729) (-4.6519, -55.5068) (-4.6457, -55.5339) (-4.6409, -55.5543) (-4.6377, -55.5678) (-4.6361, -55.5746) knots 0 0 0 0 0 0 0.01428571 0.02857143 0.04285714 0.05714286 0.07142857 0.08571429 0.1 0.11428571 0.12857143 0.14285714 0.15714286 0.17142857 0.18571429 0.2 0.21428571 0.22857143 0.24285714 0.25714286 0.27142857 0.28571429 0.3 0.31428571 0.32857143 0.34285714 0.35714286 0.37142857 0.38571429 0.4 0.41428571 0.42857143 0.44285714 0.45714286 0.47142857 0.48571429 0.5 0.51428571 0.52857143 0.54285714 0.55714286 0.57142857 0.58571429 0.6 0.61428571 0.62857143 0.64285714 0.65714286 0.67142857 0.68571429 0.7 0.71428571 0.72857143 0.74285714 0.75714286 0.77142857 0.78571429 0.8 0.81428571 0.82857143 0.84285714 0.85714286 0.87142857 0.88571429 0.9 0.91428571 0.92857143 0.94285714 0.95714286 0.97142857 0.98571429 1 1 1 1 1 1
  arc A22 (-4.6361, -55.5746) -> (-3.7723, -55.8061) centre (0, -40) ccw
  spline S11 degree 5 poles (-3.7723, -55.8061) (-3.7675, -55.801) (-3.758, -55.7908) (-3.7437, -55.7756) (-3.7248, -55.7552) (-3.7012, -55.7297) (-3.6779, -55.704) (-3.6546, -55.6784) (-3.6315, -55.6526) (-3.6086, -55.6268) (-3.5858, -55.6009) (-3.5631, -55.5749) (-3.5406, -55.5489) (-3.5183, -55.5228) (-3.4961, -55.4967) (-3.4741, -55.4704) (-3.4522, -55.4442) (-3.4304, -55.4178) (-3.4089, -55.3914) (-3.3875, -55.3649) (-3.3662, -55.3383) (-3.3451, -55.3117) (-3.3242, -55.285) (-3.3034, -55.2583) (-3.2828, -55.2315) (-3.2624, -55.2046) (-3.2421, -55.1777) (-3.222, -55.1506) (-3.2021, -55.1236) (-3.1823, -55.0964) (-3.1628, -55.0692) (-3.1434, -55.042) (-3.1241, -55.0146) (-3.1051, -54.9872) (-3.0862, -54.9597) (-3.0675, -54.9322) (-3.0491, -54.9046) (-3.0307, -54.877) (-3.0126, -54.8492) (-2.9947, -54.8214) (-2.977, -54.7936) (-2.9594, -54.7657) (-2.9421, -54.7377) (-2.925, -54.7096) (-2.9081, -54.6815) (-2.8914, -54.6533) (-2.8749, -54.625) (-2.8586, -54.5967) (-2.8425, -54.5683) (-2.8266, -54.5399) (-2.811, -54.5114) (-2.7956, -54.4828) (-2.7805, -54.4541) (-2.7656, -54.4254) (-2.751, -54.3966) (-2.7367, -54.3677) (-2.7225, -54.3387) (-2.7086, -54.3097) (-2.6949, -54.2807) (-2.6815, -54.2515) (-2.6685, -54.2223) (-2.6558, -54.193) (-2.6435, -54.1635) (-2.6317, -54.134) (-2.6202, -54.1044) (-2.609, -54.0747) (-2.5979, -54.0449) (-2.5871, -54.0152) (-2.5766, -53.9854) (-2.5667, -53.9554) (-2.5576, -53.9253) (-2.5512, -53.9009) (-2.5471, -53.8825) (-2.5447, -53.8702) (-2.5435, -53.864) knots -1 -1 -1 -1 -1 -1 -0.98571429 -0.97142857 -0.95714286 -0.94285714 -0.92857143 -0.91428571 -0.9 -0.88571429 -0.87142857 -0.85714286 -0.84285714 -0.82857143 -0.81428571 -0.8 -0.78571429 -0.77142857 -0.75714286 -0.74285714 -0.72857143 -0.71428571 -0.7 -0.68571429 -0.67142857 -0.65714286 -0.64285714 -0.62857143 -0.61428571 -0.6 -0.58571429 -0.57142857 -0.55714286 -0.54285714 -0.52857143 -0.51428571 -0.5 -0.48571429 -0.47142857 -0.45714286 -0.44285714 -0.42857143 -0.41428571 -0.4 -0.38571429 -0.37142857 -0.35714286 -0.34285714 -0.32857143 -0.31428571 -0.3 -0.28571429 -0.27142857 -0.25714286 -0.24285714 -0.22857143 -0.21428571 -0.2 -0.18571429 -0.17142857 -0.15714286 -0.14285714 -0.12857143 -0.11428571 -0.1 -0.08571429 -0.07142857 -0.05714286 -0.04285714 -0.02857143 -0.01428571 0 0 0 0 0 0
  line L11 (-2.5435, -53.864) -> (-2.4711, -53.4718)
  arc A23 (-2.1846, -53.2706) -> (-2.4711, -53.4718) centre (-2.2252, -53.5173) ccw
  arc A24 (-2.1846, -53.2706) -> (-1.3245, -53.3838) centre (0, -40) ccw
  arc A25 (-1.0999, -53.6524) -> (-1.3245, -53.3838) centre (-1.3491, -53.6326) ccw
  line L12 (-1.0999, -53.6524) -> (-1.1314, -54.0499)
  spline S12 degree 5 poles (-1.1314, -54.0499) (-1.1319, -54.0562) (-1.1327, -54.0687) (-1.1335, -54.0876) (-1.1337, -54.1127) (-1.1327, -54.1442) (-1.1308, -54.1757) (-1.1284, -54.2072) (-1.1257, -54.2388) (-1.1227, -54.2703) (-1.1196, -54.3019) (-1.1161, -54.3335) (-1.1123, -54.3651) (-1.1081, -54.3967) (-1.1035, -54.4283) (-1.0984, -54.4599) (-1.093, -54.4916) (-1.0873, -54.5232) (-1.0814, -54.5548) (-1.0752, -54.5864) (-1.0688, -54.618) (-1.0622, -54.6496) (-1.0552, -54.6812) (-1.048, -54.7128) (-1.0406, -54.7444) (-1.0329, -54.776) (-1.0249, -54.8076) (-1.0168, -54.8392) (-1.0083, -54.8708) (-0.9997, -54.9023) (-0.9909, -54.9339) (-0.9818, -54.9654) (-0.9725, -54.997) (-0.963, -55.0285) (-0.9533, -55.06) (-0.9434, -55.0915) (-0.9333, -55.123) (-0.923, -55.1545) (-0.9124, -55.1859) (-0.9017, -55.2174) (-0.8908, -55.2488) (-0.8797, -55.2802) (-0.8684, -55.3116) (-0.8569, -55.343) (-0.8452, -55.3743) (-0.8333, -55.4057) (-0.8213, -55.437) (-0.809, -55.4683) (-0.7966, -55.4996) (-0.784, -55.5309) (-0.7712, -55.5621) (-0.7583, -55.5934) (-0.7451, -55.6246) (-0.7318, -55.6558) (-0.7183, -55.6869) (-0.7047, -55.7181) (-0.6909, -55.7492) (-0.6769, -55.7803) (-0.6627, -55.8114) (-0.6484, -55.8425) (-0.6339, -55.8735) (-0.6192, -55.9045) (-0.6044, -55.9355) (-0.5894, -55.9664) (-0.5742, -55.9974) (-0.5589, -56.0283) (-0.5434, -56.0592) (-0.5278, -56.09) (-0.512, -56.1208) (-0.496, -56.1516) (-0.4799, -56.1824) (-0.4669, -56.207) (-0.4571, -56.2254) (-0.4505, -56.2377) (-0.4472, -56.2438) knots 0 0 0 0 0 0 0.01428571 0.02857143 0.04285714 0.05714286 0.07142857 0.08571429 0.1 0.11428571 0.12857143 0.14285714 0.15714286 0.17142857 0.18571429 0.2 0.21428571 0.22857143 0.24285714 0.25714286 0.27142857 0.28571429 0.3 0.31428571 0.32857143 0.34285714 0.35714286 0.37142857 0.38571429 0.4 0.41428571 0.42857143 0.44285714 0.45714286 0.47142857 0.48571429 0.5 0.51428571 0.52857143 0.54285714 0.55714286 0.57142857 0.58571429 0.6 0.61428571 0.62857143 0.64285714 0.65714286 0.67142857 0.68571429 0.7 0.71428571 0.72857143 0.74285714 0.75714286 0.77142857 0.78571429 0.8 0.81428571 0.82857143 0.84285714 0.85714286 0.87142857 0.88571429 0.9 0.91428571 0.92857143 0.94285714 0.95714286 0.97142857 0.98571429 1 1 1 1 1 1
  arc A26 (-0.4472, -56.2438) -> (0.4472, -56.2438) centre (0, -40) ccw
  spline S13 degree 5 poles (0.4472, -56.2438) (0.4505, -56.2377) (0.4571, -56.2254) (0.4669, -56.207) (0.4799, -56.1824) (0.496, -56.1516) (0.512, -56.1208) (0.5278, -56.09) (0.5434, -56.0592) (0.5589, -56.0283) (0.5742, -55.9974) (0.5894, -55.9664) (0.6044, -55.9355) (0.6192, -55.9045) (0.6339, -55.8735) (0.6484, -55.8425) (0.6627, -55.8114) (0.6769, -55.7803) (0.6909, -55.7492) (0.7047, -55.7181) (0.7183, -55.6869) (0.7318, -55.6558) (0.7451, -55.6246) (0.7583, -55.5934) (0.7712, -55.5621) (0.784, -55.5309) (0.7966, -55.4996) (0.809, -55.4683) (0.8213, -55.437) (0.8333, -55.4057) (0.8452, -55.3743) (0.8569, -55.343) (0.8684, -55.3116) (0.8797, -55.2802) (0.8908, -55.2488) (0.9017, -55.2174) (0.9124, -55.1859) (0.923, -55.1545) (0.9333, -55.123) (0.9434, -55.0915) (0.9533, -55.06) (0.963, -55.0285) (0.9725, -54.997) (0.9818, -54.9654) (0.9909, -54.9339) (0.9997, -54.9023) (1.0083, -54.8708) (1.0168, -54.8392) (1.0249, -54.8076) (1.0329, -54.776) (1.0406, -54.7444) (1.048, -54.7128) (1.0552, -54.6812) (1.0622, -54.6496) (1.0688, -54.618) (1.0752, -54.5864) (1.0814, -54.5548) (1.0873, -54.5232) (1.093, -54.4916) (1.0984, -54.4599) (1.1035, -54.4283) (1.1081, -54.3967) (1.1123, -54.3651) (1.1161, -54.3335) (1.1196, -54.3019) (1.1227, -54.2703) (1.1257, -54.2388) (1.1284, -54.2072) (1.1308, -54.1757) (1.1327, -54.1442) (1.1337, -54.1127) (1.1335, -54.0876) (1.1327, -54.0687) (1.1319, -54.0562) (1.1314, -54.0499) knots -1 -1 -1 -1 -1 -1 -0.98571429 -0.97142857 -0.95714286 -0.94285714 -0.92857143 -0.91428571 -0.9 -0.88571429 -0.87142857 -0.85714286 -0.84285714 -0.82857143 -0.81428571 -0.8 -0.78571429 -0.77142857 -0.75714286 -0.74285714 -0.72857143 -0.71428571 -0.7 -0.68571429 -0.67142857 -0.65714286 -0.64285714 -0.62857143 -0.61428571 -0.6 -0.58571429 -0.57142857 -0.55714286 -0.54285714 -0.52857143 -0.51428571 -0.5 -0.48571429 -0.47142857 -0.45714286 -0.44285714 -0.42857143 -0.41428571 -0.4 -0.38571429 -0.37142857 -0.35714286 -0.34285714 -0.32857143 -0.31428571 -0.3 -0.28571429 -0.27142857 -0.25714286 -0.24285714 -0.22857143 -0.21428571 -0.2 -0.18571429 -0.17142857 -0.15714286 -0.14285714 -0.12857143 -0.11428571 -0.1 -0.08571429 -0.07142857 -0.05714286 -0.04285714 -0.02857143 -0.01428571 0 0 0 0 0 0
  line L13 (1.1314, -54.0499) -> (1.0999, -53.6524)
  arc A27 (1.3245, -53.3838) -> (1.0999, -53.6524) centre (1.3491, -53.6326) ccw
  arc A28 (1.3245, -53.3838) -> (2.1846, -53.2706) centre (0, -40) ccw
  arc A29 (2.4711, -53.4718) -> (2.1846, -53.2706) centre (2.2252, -53.5173) ccw
  line L14 (2.4711, -53.4718) -> (2.5435, -53.864)
  spline S14 degree 5 poles (2.5435, -53.864) (2.5447, -53.8702) (2.5471, -53.8825) (2.5512, -53.9009) (2.5576, -53.9253) (2.5667, -53.9554) (2.5766, -53.9854) (2.5871, -54.0152) (2.5979, -54.0449) (2.609, -54.0747) (2.6202, -54.1044) (2.6317, -54.134) (2.6435, -54.1635) (2.6558, -54.193) (2.6685, -54.2223) (2.6815, -54.2515) (2.6949, -54.2807) (2.7086, -54.3097) (2.7225, -54.3387) (2.7367, -54.3677) (2.751, -54.3966) (2.7656, -54.4254) (2.7805, -54.4541) (2.7956, -54.4828) (2.811, -54.5114) (2.8266, -54.5399) (2.8425, -54.5683) (2.8586, -54.5967) (2.8749, -54.625) (2.8914, -54.6533) (2.9081, -54.6815) (2.925, -54.7096) (2.9421, -54.7377) (2.9594, -54.7657) (2.977, -54.7936) (2.9947, -54.8214) (3.0126, -54.8492) (3.0307, -54.877) (3.0491, -54.9046) (3.0675, -54.9322) (3.0862, -54.9597) (3.1051, -54.9872) (3.1241, -55.0146) (3.1434, -55.042) (3.1628, -55.0692) (3.1823, -55.0964) (3.2021, -55.1236) (3.222, -55.1506) (3.2421, -55.1777) (3.2624, -55.2046) (3.2828, -55.2315) (3.3034, -55.2583) (3.3242, -55.285) (3.3451, -55.3117) (3.3662, -55.3383) (3.3875, -55.3649) (3.4089, -55.3914) (3.4304, -55.4178) (3.4522, -55.4442) (3.4741, -55.4704) (3.4961, -55.4967) (3.5183, -55.5228) (3.5406, -55.5489) (3.5631, -55.5749) (3.5858, -55.6009) (3.6086, -55.6268) (3.6315, -55.6526) (3.6546, -55.6784) (3.6779, -55.704) (3.7012, -55.7297) (3.7248, -55.7552) (3.7437, -55.7756) (3.758, -55.7908) (3.7675, -55.801) (3.7723, -55.8061) knots 0 0 0 0 0 0 0.01428571 0.02857143 0.04285714 0.05714286 0.07142857 0.08571429 0.1 0.11428571 0.12857143 0.14285714 0.15714286 0.17142857 0.18571429 0.2 0.21428571 0.22857143 0.24285714 0.25714286 0.27142857 0.28571429 0.3 0.31428571 0.32857143 0.34285714 0.35714286 0.37142857 0.38571429 0.4 0.41428571 0.42857143 0.44285714 0.45714286 0.47142857 0.48571429 0.5 0.51428571 0.52857143 0.54285714 0.55714286 0.57142857 0.58571429 0.6 0.61428571 0.62857143 0.64285714 0.65714286 0.67142857 0.68571429 0.7 0.71428571 0.72857143 0.74285714 0.75714286 0.77142857 0.78571429 0.8 0.81428571 0.82857143 0.84285714 0.85714286 0.87142857 0.88571429 0.9 0.91428571 0.92857143 0.94285714 0.95714286 0.97142857 0.98571429 1 1 1 1 1 1
  arc A30 (3.7723, -55.8061) -> (4.6361, -55.5746) centre (0, -40) ccw
  spline S15 degree 5 poles (4.6361, -55.5746) (4.6377, -55.5678) (4.6409, -55.5543) (4.6457, -55.5339) (4.6519, -55.5068) (4.6595, -55.4729) (4.6669, -55.439) (4.6742, -55.4052) (4.6813, -55.3713) (4.6883, -55.3375) (4.6951, -55.3037) (4.7017, -55.2699) (4.7082, -55.2361) (4.7145, -55.2023) (4.7206, -55.1686) (4.7266, -55.1348) (4.7324, -55.1011) (4.738, -55.0674) (4.7435, -55.0338) (4.7488, -55.0001) (4.754, -54.9665) (4.7589, -54.9329) (4.7637, -54.8993) (4.7683, -54.8658) (4.7727, -54.8323) (4.777, -54.7988) (4.7811, -54.7653) (4.785, -54.7319) (4.7887, -54.6984) (4.7922, -54.6651) (4.7956, -54.6317) (4.7987, -54.5984) (4.8017, -54.5651) (4.8045, -54.5319) (4.8071, -54.4986) (4.8095, -54.4655) (4.8118, -54.4323) (4.8138, -54.3992) (4.8156, -54.3661) (4.8172, -54.3331) (4.8187, -54.3001) (4.8199, -54.2672) (4.8209, -54.2342) (4.8217, -54.2014) (4.8223, -54.1686) (4.8227, -54.1358) (4.8228, -54.1031) (4.8228, -54.0704) (4.8225, -54.0378) (4.822, -54.0052) (4.8213, -53.9727) (4.8203, -53.9403) (4.8191, -53.9079) (4.8176, -53.8756) (4.8158, -53.8433) (4.8138, -53.8111) (4.8116, -53.779) (4.8092, -53.7469) (4.8065, -53.7149) (4.8035, -53.6829) (4.8002, -53.6511) (4.7965, -53.6194) (4.7924, -53.5877) (4.7879, -53.5562) (4.783, -53.5248) (4.7779, -53.4935) (4.7726, -53.4623) (4.7671, -53.4311) (4.7613, -53.4) (4.7549, -53.3691) (4.7477, -53.3384) (4.741, -53.3142) (4.7354, -53.2962) (4.7313, -53.2843) (4.7292, -53.2783) knots -1 -1 -1 -1 -1 -1 -0.98571429 -0.97142857 -0.95714286 -0.94285714 -0.92857143 -0.91428571 -0.9 -0.88571429 -0.87142857 -0.85714286 -0.84285714 -0.82857143 -0.81428571 -0.8 -0.78571429 -0.77142857 -0.75714286 -0.74285714 -0.72857143 -0.71428571 -0.7 -0.68571429 -0.67142857 -0.65714286 -0.64285714 -0.62857143 -0.61428571 -0.6 -0.58571429 -0.57142857 -0.55714286 -0.54285714 -0.52857143 -0.51428571 -0.5 -0.48571429 -0.47142857 -0.45714286 -0.44285714 -0.42857143 -0.41428571 -0.4 -0.38571429 -0.37142857 -0.35714286 -0.34285714 -0.32857143 -0.31428571 -0.3 -0.28571429 -0.27142857 -0.25714286 -0.24285714 -0.22857143 -0.21428571 -0.2 -0.18571429 -0.17142857 -0.15714286 -0.14285714 -0.12857143 -0.11428571 -0.1 -0.08571429 -0.07142857 -0.05714286 -0.04285714 -0.02857143 -0.01428571 0 0 0 0 0 0
  line L15 (4.7292, -53.2783) -> (4.5959, -52.9025)
  arc A31 (4.7433, -52.585) -> (4.5959, -52.9025) centre (4.8315, -52.8189) ccw
  arc A32 (4.7433, -52.585) -> (5.5449, -52.253) centre (0, -40) ccw
  arc A33 (5.8737, -52.3732) -> (5.5449, -52.253) centre (5.648, -52.4807) ccw
  line L16 (5.8737, -52.3732) -> (6.0451, -52.7333)
  spline S16 degree 5 poles (6.0451, -52.7333) (6.0478, -52.739) (6.0534, -52.7503) (6.0621, -52.767) (6.0745, -52.7888) (6.0911, -52.8156) (6.1085, -52.8419) (6.1264, -52.868) (6.1445, -52.894) (6.1629, -52.9198) (6.1814, -52.9456) (6.2002, -52.9713) (6.2193, -52.9967) (6.2387, -53.022) (6.2585, -53.047) (6.2787, -53.0719) (6.2992, -53.0966) (6.3199, -53.1211) (6.3409, -53.1455) (6.362, -53.1698) (6.3834, -53.194) (6.405, -53.218) (6.4268, -53.2419) (6.4488, -53.2657) (6.471, -53.2894) (6.4935, -53.3129) (6.5162, -53.3362) (6.5391, -53.3595) (6.5621, -53.3826) (6.5854, -53.4057) (6.6088, -53.4286) (6.6324, -53.4514) (6.6562, -53.474) (6.6802, -53.4966) (6.7044, -53.519) (6.7287, -53.5413) (6.7532, -53.5635) (6.7779, -53.5856) (6.8028, -53.6076) (6.8278, -53.6295) (6.8529, -53.6512) (6.8783, -53.6729) (6.9038, -53.6944) (6.9294, -53.7158) (6.9552, -53.7372) (6.9812, -53.7584) (7.0073, -53.7795) (7.0335, -53.8005) (7.0599, -53.8214) (7.0865, -53.8422) (7.1132, -53.8628) (7.14, -53.8834) (7.167, -53.9039) (7.1941, -53.9242) (7.2214, -53.9445) (7.2488, -53.9646) (7.2763, -53.9847) (7.304, -54.0046) (7.3318, -54.0244) (7.3597, -54.0442) (7.3878, -54.0638) (7.416, -54.0833) (7.4443, -54.1027) (7.4728, -54.122) (7.5014, -54.1412) (7.5301, -54.1603) (7.559, -54.1793) (7.5879, -54.1982) (7.617, -54.217) (7.6463, -54.2357) (7.6756, -54.2543) (7.6992, -54.2691) (7.7169, -54.2802) (7.7287, -54.2875) (7.7347, -54.2912) knots 0 0 0 0 0 0 0.01428571 0.02857143 0.04285714 0.05714286 0.07142857 0.08571429 0.1 0.11428571 0.12857143 0.14285714 0.15714286 0.17142857 0.18571429 0.2 0.21428571 0.22857143 0.24285714 0.25714286 0.27142857 0.28571429 0.3 0.31428571 0.32857143 0.34285714 0.35714286 0.37142857 0.38571429 0.4 0.41428571 0.42857143 0.44285714 0.45714286 0.47142857 0.48571429 0.5 0.51428571 0.52857143 0.54285714 0.55714286 0.57142857 0.58571429 0.6 0.61428571 0.62857143 0.64285714 0.65714286 0.67142857 0.68571429 0.7 0.71428571 0.72857143 0.74285714 0.75714286 0.77142857 0.78571429 0.8 0.81428571 0.82857143 0.84285714 0.85714286 0.87142857 0.88571429 0.9 0.91428571 0.92857143 0.94285714 0.95714286 0.97142857 0.98571429 1 1 1 1 1 1
  arc A34 (7.7347, -54.2912) -> (8.5092, -53.844) centre (0, -40) ccw